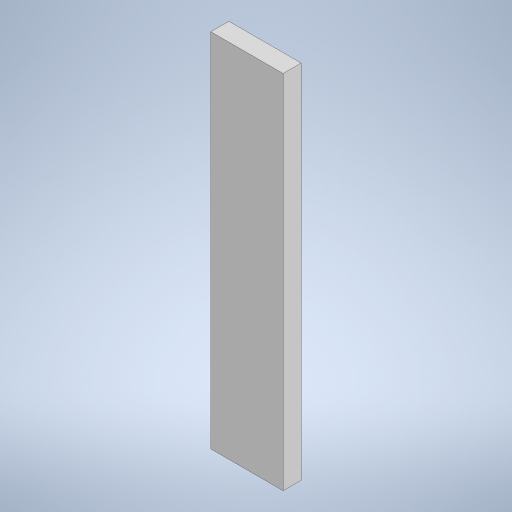
# Autodesk Inventor part: Linear_guide
Saved by Autodesk Inventor 2024.3 (Build 283343000, 343)
## iProperties
Created: 2025-09-03
Part Number: Linear_guide
Material: Generico
Document SubType Name: Modeling
Designer: chris
Density: 1 g/cm^3
Appearance: Default
Author: chris
Autodesk Inventor part; units mm, degrees
ref_plane "YZ Plane" through (0, 0, 0) normal (1, 0, 0) x (0, 1, 0)
ref_plane "XZ Plane" through (0, 0, 0) normal (0, 1, 0) x (-1, 0, 0)
ref_plane "XY Plane" through (0, 0, 0) normal (0, 0, 1) x (1, 0, 0)
sketch "Schizzo1" plane through (0, 0, 0) normal (0, 0, 1) x (1, 0, 0)
  line L0 (0.2, 1) -> (-0.2, 1)
  line L1 (-0.2, 1) -> (-0.2, -1)
  line L2 (-0.2, -1) -> (0.2, -1)
  line L3 (0.2, -1) -> (0.2, 1)
  line L4 (0.2, 1) -> (-0.2, -1) construction
  line L5 (-0.2, 1) -> (0.2, -1) construction
  point P0 (0, 0)
  dimension "d0" = 0.4
  dimension "d1" = 2
  constraints: 12 end point, 2 midpoint, 2 parallel, 1 horizontal, 1 perpendicular
  measures "d0" distance of L1.end L2.end
  measures "d1" distance of L0.end L1.end
extrude "Estrusione1" add sketch "Schizzo1" along normal blind 0.1
